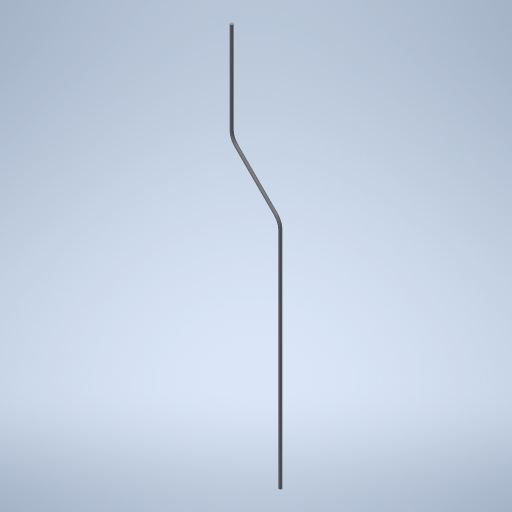
# Autodesk Inventor part: cable indice
Saved by Autodesk Inventor 2023 (Build 270158000, 158)
## iProperties
Created: 2022-10-18
Part Number: cable indice
Material: Generic
Document SubType Name: Modeling
Designer: Xiaba
Density: 1 g/cm^3
Appearance: Default
Author: Xiaba
Autodesk Inventor part; units mm, degrees
ref_plane "YZ Plane" through (0, 0, 0) normal (1, 0, 0) x (0, 1, 0)
ref_plane "XZ Plane" through (0, 0, 0) normal (0, 1, 0) x (-1, 0, 0)
ref_plane "XY Plane" through (0, 0, 0) normal (0, 0, 1) x (1, 0, 0)
sketch "Sketch1" plane through (0, 0, 0) normal (0, 1, 0) x (-1, 0, 0)
  circle A0 centre (0, 0) radius 0.45
  dimension "d0" = 0.9
  constraints: 1 centre point, 1 coincident
  measures "d0" diameter of A0
sketch "Sketch2" plane through (0, 0, 0) normal (0, 0, 1) x (1, 0, 0)
  line L0 (0, 0) -> (0, 0.1)
  line L1 (0, 0.1) -> (0, 68.0289)
  line L2 (0, 70.1) -> (-27.343, 70.1) construction
  line L3 (-1.4645, 71.5645) -> (-13.3848, 83.4848)
  line L4 (-14.8492, 87.0203) -> (-14.8492, 114.9492)
  arc A0 (-14.8492, 87.0203) -> (-13.3848, 83.4848) centre (-9.8492, 87.0203) ccw
  arc A1 (0, 68.0289) -> (-1.4645, 71.5645) centre (-5, 68.0289) ccw
  point P0 (-14.8492, 84.9492)
  dimension "d1" = 0.1
  dimension "d4" = 70
  dimension "d5" = 45
  dimension "d6" = 21
  dimension "d7" = 30
  dimension "d8" = 5
  dimension "d9" = 5
  constraints: 10 end point, 4 point on circle, 4 point on line, 4 tangent, 3 vertical, 2 centre point, 1 horizontal
  measures "d1" distance of L0.start L0.end
  measures "d4" distance of L0.end L2.start
  measures "d5" angle of L2 L3
  measures "d6" distance of L2.start point (-14.849, 84.949)
  measures "d7" distance of point (-14.849, 84.949) L4.end
  measures "d8" radius of A0
  measures "d9" radius of A1
sweep "Sweep2" add profiles "Sketch1" path "Sketch2"
body "Solid2"
